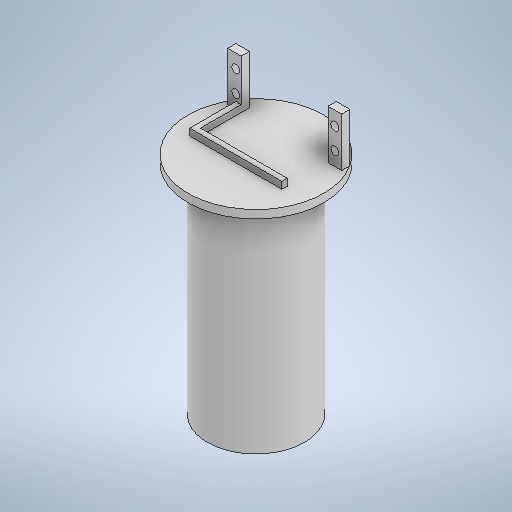
# Autodesk Inventor part: 零件3
Saved by Autodesk Inventor 2025 (Build 290162000, 162)
## iProperties
Created: 2024-03-30
Part Number: 零件3
Material: 常规
Document SubType Name: Modeling
Designer: Huijun Wang
Density: 1 g/cm^3
Appearance: 默认
Author: Huijun Wang
Autodesk Inventor part; units mm, degrees
ref_plane "YZ Plane" through (0, 0, 0) normal (1, 0, 0) x (0, 1, 0)
ref_plane "XZ Plane" through (0, 0, 0) normal (0, 1, 0) x (-1, 0, 0)
ref_plane "XY Plane" through (0, 0, 0) normal (0, 0, 1) x (1, 0, 0)
sketch "草图1" plane through (0, 0, 0) normal (0, 1, 0) x (-1, 0, 0)
  circle A0 centre (0, 0) radius 17.907692
  constraints: 1 centre point
extrude "拉伸1" add sketch "草图1" along normal blind 80
sketch "草图6" plane through (0, 0, 0) normal (0, -1, 0) x (1, 0, 0)
  line L0 (0, 0) -> (0, -13.5)
  line L1 (0, -13.5) -> (10, -13.5)
  line L2 (10, -13.5) -> (10, 13.5)
  line L3 (10, 13.5) -> (-10, 13.5)
  line L4 (-10, 13.5) -> (-10, -13.5)
  line L5 (-10, -13.5) -> (0, -13.5)
  dimension "d56" = 10
  dimension "d63" = 20
  dimension "d64" = 27
  constraints: 12 end point, 5 perpendicular, 1 point on line, 1 vertical
  measures "d56" distance of L0.end L1.end
  measures "d63" distance of L2.end L3.end
  measures "d64" distance of L3.end L4.end
sketch "草图7" plane through (0, 0, 0) normal (0, -1, 0) x (1, 0, 0)
  line L0 (0, 0) -> (0, -9.594248)
  line L1 (0, 0) -> (0, -10)
  line L2 (0, 0) -> (0, -6)
  line L3 (0, -6) -> (4.5, -6)
  line L4 (4.5, 6) -> (-4.5, 6)
  line L5 (-4.5, 6) -> (-4.5, -6)
  line L6 (0, 0) -> (0, 10)
  circle A0 centre (4.5, 6) radius 1.5
  circle A1 centre (4.5, -6) radius 1.5
  circle A2 centre (-4.5, -6) radius 1.5
  circle A3 centre (0, -10) radius 1.5
  circle A4 centre (0, 10) radius 1.5
  circle A5 centre (-4.5, 6) radius 1.5
  dimension "d76" = 6
  dimension "d77" = 12
  dimension "d78" = 3
  dimension "d79" = 3
  dimension "d80" = 10
  dimension "d81" = 4.5
  dimension "d85" = 4.5
  dimension "d86" = 3
  dimension "d87" = 3
  dimension "d88" = 3
  dimension "d89" = 3
  dimension "d90" = 10
  dimension "d91" = 4.5
  dimension "d92" = 6
  dimension "d93" = 4.5
  constraints: 14 end point, 8 coincident, 6 centre point, 3 point on line, 2 vertical, 1 perpendicular
  measures "d76" distance of L2.start L3.start
  measures "d77" distance of L5.start L5.end
  measures "d78" diameter of A2
  measures "d79" diameter of A4
  measures "d80" distance of point (0, 0) L6.end
  measures "d81" horizontal distance of L3.end point (0, 0)
  measures "d85" distance from line of L5 point (0, 0)
  measures "d86" diameter of A0
  measures "d87" diameter of A5
  measures "d88" diameter of A1
  measures "d89" diameter of A3
  measures "d90" distance of L1.end point (0, 0)
  measures "d91" horizontal distance of L5.end point (0, 0)
  measures "d92" vertical distance of point (0, 0) L4.start
  measures "d93" horizontal distance of point (0, 0) L4.start
extrude "拉伸2" cut sketch "草图7" against normal blind 42
extrude "拉伸3" cut sketch "草图6" against normal blind 2
sketch "草图8" plane through (0, 80, 0) normal (0, 1, 0) x (1, 0, 0)
  circle A0 centre (0, 0) radius 17.907692
  circle A1 centre (0, 0) radius 25
  line L0 (-21, 13.56466) -> (21, 13.56466)
  line L1 (-21, 13.56466) -> (-21, 10.56466)
  line L2 (-21, 10.56466) -> (-16, 10.56466)
  line L3 (21, 13.56466) -> (21, 10.56466)
  line L4 (21, 10.56466) -> (16, 10.56466)
  line L5 (-21, 10.56466) -> (-16, 10.56466)
  line L6 (-16, 10.56466) -> (-16, 13.56466)
  line L7 (21, 10.56466) -> (16, 10.56466)
  line L8 (16, 10.56466) -> (16, 13.56466)
  line L9 (16, 10.56466) -> (16, 13.56466)
  line L10 (21, 13.56466) -> (21, 10.56466)
  line L11 (16, 10.56466) -> (21, 10.56466)
  line L12 (21, 13.56466) -> (16, 13.56466)
  dimension "d99" = 50
  dimension "d100" = 42
  dimension "d101" = 3
  dimension "d109" = 5
  dimension "d129" = 5
  constraints: 26 end point, 4 perpendicular, 3 collinear, 3 point on line, 2 horizontal, 2 point on circle, 2 vertical, 1 centre point, 1 coincident, 1 parallel
  measures "d99" diameter of A1
  measures "d100" distance of L0.start L0.end
  measures "d101" distance of L0.start L1.end
  measures "d109" distance of L1.end L5.end
  measures "d129" distance between parallel lines of L3 L8
sketch "草图9" plane through (0, 80, 0) normal (0, 1, 0) x (1, 0, 0)
  circle A0 centre (0, 0) radius 25
  line L0 (-21, 13.56466) -> (-16, 13.56466)
  line L1 (-16, 10.56466) -> (-21, 10.56466)
  line L2 (-21, 10.56466) -> (-21, 13.56466)
  line L3 (16, 13.56466) -> (21, 13.56466)
  line L4 (21, 10.56466) -> (16, 10.56466)
  line L5 (-21, 13.56466) -> (-15, 13.56466)
  line L6 (-15, 13.56466) -> (-15, 10.56466)
  line L7 (-15, 10.56466) -> (-21, 10.56466)
  line L8 (21, 13.56466) -> (15, 13.56466)
  line L9 (15, 13.56466) -> (15, 10.56466)
  line L10 (15, 10.56466) -> (21, 10.56466)
  line L11 (21, 10.56466) -> (15, 10.56466)
  dimension "d105" = 3
  dimension "d106" = 6
  dimension "d107" = 6
  dimension "d108" = 3
  constraints: 24 end point, 5 point on line, 3 horizontal, 3 perpendicular, 2 collinear, 2 point on circle, 1 centre point, 1 coincident
  measures "d105" distance of L0.end L1.start
  measures "d106" distance of L0.start L5.end
  measures "d107" distance of L3.end L8.end
  measures "d108" distance of L8.end L9.end
sketch "草图9 outline for 拉伸4" plane through (0, 80, 0) normal (0, 1, 0) x (1, 0, 0)
  circle A0 centre (0, 0) radius 25
extrude "拉伸4" add sketch "草图9 outline for 拉伸4" along normal blind 3
extrude "拉伸5" add sketch "草图8" along normal blind 21 contours L0 L3 L4 L8 | L6 L2 L1 L0
sketch "草图10" plane through (21, 83, -13.56466) normal (0, 0, -1) x (-1, 0, 0)
  line L0 (0, 0) -> (5, 0) projected
  line L1 (0, 0) -> (2.5, 0)
  line L2 (2.5, 0) -> (2.5, 5)
  circle A0 centre (2.5, 5) radius 1.5
  line L3 (2.5, 5) -> (2.5, 5.79)
  line L4 (2.5, 5) -> (2.5, 12.9)
  circle A1 centre (2.5, 12.9) radius 1.5
  line L5 (42, 0) -> (37, 0) projected
  line L6 (37, 0) -> (39.5, 0)
  line L7 (39, 5) -> (39, 12.9)
  circle A2 centre (39, 12.9) radius 1.5
  circle A3 centre (39, 5) radius 1.5
  point P0 (21, -83)
  dimension "d115" = 3
  dimension "d116" = 0.79
  dimension "d117" = 7.9
  dimension "d118" = 3
  dimension "d119" = 3
  dimension "d120" = 3
  constraints: 12 end point, 4 centre point, 4 coincident, 4 vertical, 2 midpoint
  measures "d115" diameter of A0
  measures "d116" distance of L3.start L3.end
  measures "d117" distance of L3.start L4.end
  measures "d118" diameter of A1
  measures "d119" diameter of A2
  measures "d120" diameter of A3
extrude "拉伸6" cut sketch "草图10" against normal blind 3
sketch "草图11" plane through (0, 83, 0) normal (0, 1, 0) x (1, 0, 0)
  line L0 (-22, 10.56466) -> (-16, 10.56466)
  line L1 (-16, 10.56466) -> (-16, -4.43534)
  line L2 (-16, -4.43534) -> (-18, -4.43534)
  line L3 (-18, -4.43534) -> (-18, 10.56466)
  line L4 (-16, -4.43534) -> (-16, -6.43534)
  line L5 (-16, -6.43534) -> (16, -6.43534)
  line L6 (16, -6.43534) -> (16, -4.43534)
  line L7 (16, -4.43534) -> (-16, -4.43534)
  line L8 (-16, -6.43534) -> (-18, -6.43534)
  line L9 (-18, -6.43534) -> (-18, -4.43534)
  line L10 (-16, 10.56466) -> (-18, 10.56466)
  line L11 (0, 0) -> (0, -28) construction
  dimension "d123" = 15
  dimension "d124" = 2
  dimension "d125" = 2
  dimension "d126" = 32
  constraints: 24 end point, 5 vertical, 2 point on line, 1 other
  measures "d123" distance of L0.end L1.end
  measures "d124" distance of L1.end L2.end
  measures "d125" distance of L1.end L4.end
  measures "d126" distance of L4.end L5.end
extrude "拉伸7" add sketch "草图11" along normal blind 2.5
